Autodesk Fusion 360 part; units mm, degrees
(part 2 of 2)
sketch "SDVX Layout" plane through (0, 77, 0) normal (0, 1, 0) x (-1, 0, 0)
  circle A0 centre (-230, 0) radius 2.5
  circle A1 centre (230, 110) radius 2.5
  circle A2 centre (-230, -110) radius 2.5
  circle A3 centre (-230, 110) radius 2.5
  circle A4 centre (0, 110) radius 2.5
  circle A5 centre (230, -110) radius 2.5
  circle A6 centre (0, -110) radius 2.5
  circle A7 centre (230, 0) radius 2.5
  line L0 (-248, 128) -> (-248, -128)
  line L1 (-248, -128) -> (248, -128)
  line L2 (248, -128) -> (248, 128)
  line L3 (248, 128) -> (-248, 128)
  line L4 (248, 0) -> (-248, 0) construction
  line L5 (-151.5, -36) -> (151.5, -36)
  line L6 (67, 28.5) -> (67, -28.5)
  line L7 (-54.5, 62.5) -> (-100.5, 62.5)
  line L8 (-84.5, 31) -> (-146.5, 31) construction
  circle A8 centre (192.49, -61.5) radius 1.75
  circle A9 centre (-179.5, -39) radius 1.75
  line L9 (-47.5, 55.5) -> (-107.5, 98.5) construction
  circle A10 centre (179.5, -54) radius 15 construction
  circle A11 centre (179.5, -54) radius 10
  circle A12 centre (179.5, -54) radius 20
  line L10 (144, -28.5) -> (87, -28.5)
  line L11 (107.5, 55.5) -> (107.5, 98.5)
  line L12 (144, 28.5) -> (144, -28.5)
  line L13 (69.5, -31) -> (69.5, 31) construction
  line L14 (-87, 0) -> (-144, 0) construction
  line L15 (84.5, -31) -> (146.5, 31) construction
  line L16 (-107.5, 55.5) -> (-47.5, 55.5)
  line L17 (146.5, -31) -> (84.5, 31) construction
  line L18 (-54.5, 77) -> (-100.5, 77) construction
  line L19 (67, 0) -> (87, 0) construction
  line L20 (87, 28.5) -> (144, 28.5)
  line L21 (-52.5, 60.5) -> (-102.5, 93.5) construction
  circle A13 centre (179.5, -39) radius 1.75
  line L22 (47.5, 55.5) -> (107.5, 55.5)
  line L23 (144, 0) -> (87, 0) construction
  line L24 (151.5, -36) -> (151.5, 36)
  line L25 (-87, -28.5) -> (-144, -28.5)
  circle A14 centre (-192.49, -61.5) radius 1.75
  circle A15 centre (166.51, -61.5) radius 1.75
  line L26 (84.5, -31) -> (146.5, -31) construction
  line L27 (-84.5, -31) -> (-84.5, 31) construction
  line L28 (52.5, 93.5) -> (52.5, 60.5) construction
  circle A16 centre (-179.5, -54) radius 15 construction
  line L29 (107.5, 98.5) -> (47.5, 98.5)
  line L30 (-47.5, 98.5) -> (-107.5, 98.5)
  line L31 (-102.5, 60.5) -> (-52.5, 60.5) construction
  line L32 (-102.5, 60.5) -> (-52.5, 93.5) construction
  line L33 (-100.5, 62.5) -> (-100.5, 91.5)
  line L34 (100.5, 91.5) -> (100.5, 62.5)
  line L35 (-146.5, 31) -> (-146.5, -31) construction
  line L36 (54.5, 62.5) -> (54.5, 91.5)
  line L37 (52.5, 60.5) -> (102.5, 93.5) construction
  line L38 (-146.5, -31) -> (-84.5, 31) construction
  circle A17 centre (-179.5, -54) radius 10
  line L39 (-146.5, -31) -> (-84.5, -31) construction
  line L40 (47.5, 55.5) -> (107.5, 98.5) construction
  line L41 (107.5, 55.5) -> (47.5, 98.5) construction
  line L42 (-115.5, -28.5) -> (-115.5, 28.5) construction
  line L43 (-84.5, -31) -> (-146.5, 31) construction
  circle A18 centre (-179.5, -54) radius 20
  line L44 (-144, 28.5) -> (-87, 28.5)
  line L45 (54.5, 91.5) -> (100.5, 91.5)
  line L46 (100.5, 62.5) -> (54.5, 62.5)
  line L47 (102.5, 93.5) -> (52.5, 93.5) construction
  line L48 (77.5, 62.5) -> (77.5, 91.5) construction
  line L49 (100.5, 77) -> (54.5, 77) construction
  line L50 (146.5, 31) -> (84.5, 31) construction
  line L51 (-151.5, 36) -> (-151.5, -36)
  line L52 (-107.5, 98.5) -> (-107.5, 55.5)
  line L53 (102.5, 60.5) -> (102.5, 93.5) construction
  circle A19 centre (-166.51, -61.5) radius 1.75
  line L54 (-144, -28.5) -> (-144, 28.5)
  line L55 (-102.5, 93.5) -> (-102.5, 60.5) construction
  line L56 (-87, 28.5) -> (-87, -28.5)
  line L57 (102.5, 60.5) -> (52.5, 93.5) construction
  line L58 (47.5, 98.5) -> (47.5, 55.5)
  line L59 (52.5, 60.5) -> (102.5, 60.5) construction
  line L60 (-10, 0) -> (-67, 0) construction
  line L61 (-7.5, -31) -> (-7.5, 31) construction
  line L62 (7.5, -31) -> (69.5, -31) construction
  line L63 (115.5, -28.5) -> (115.5, 28.5) construction
  line L64 (-100.5, 91.5) -> (-54.5, 91.5)
  line L65 (84.5, 31) -> (84.5, -31) construction
  line L66 (87, -28.5) -> (87, 28.5)
  line L67 (-107.5, 55.5) -> (-47.5, 98.5) construction
  line L68 (38.5, -28.5) -> (38.5, 28.5) construction
  line L69 (146.5, -31) -> (146.5, 31) construction
  line L70 (-87, 0) -> (-67, 0) construction
  line L71 (67, 0) -> (10, 0) construction
  line L72 (151.5, 36) -> (-151.5, 36)
  line L73 (67, -28.5) -> (10, -28.5)
  line L74 (151.5, -36) -> (-151.5, 36) construction
  line L75 (-151.5, -36) -> (151.5, 36) construction
  line L76 (-52.5, 93.5) -> (-102.5, 93.5) construction
  line L77 (52.5, 77) -> (-52.5, 77) construction
  line L78 (10, 28.5) -> (67, 28.5)
  line L79 (-7.5, -31) -> (-69.5, 31) construction
  line L80 (-67, 28.5) -> (-10, 28.5)
  line L81 (7.5, -31) -> (69.5, 31) construction
  line L82 (-47.5, 55.5) -> (-47.5, 98.5)
  line L83 (10, -28.5) -> (10, 28.5)
  line L84 (-7.5, 31) -> (-69.5, 31) construction
  line L85 (-69.5, -31) -> (-7.5, -31) construction
  line L86 (-67, -28.5) -> (-67, 28.5)
  line L87 (-69.5, 31) -> (-69.5, -31) construction
  line L88 (-69.5, -31) -> (-7.5, 31) construction
  line L89 (-10, 28.5) -> (-10, -28.5)
  line L90 (10, 0) -> (-10, 0) construction
  line L91 (-77.5, 62.5) -> (-77.5, 91.5) construction
  line L92 (-52.5, 60.5) -> (-52.5, 93.5) construction
  line L93 (7.5, 31) -> (7.5, -31) construction
  line L94 (-38.5, -28.5) -> (-38.5, 28.5) construction
  circle A20 centre (208, -108) radius 2.5
  line L95 (-10, -28.5) -> (-67, -28.5)
  line L96 (-54.5, 91.5) -> (-54.5, 62.5)
  line L97 (69.5, 31) -> (7.5, 31) construction
  line L98 (69.5, -31) -> (7.5, 31) construction
  line L99 (0, -96.3345) -> (23.3345, -73)
  line L100 (23.3345, -73) -> (0, -49.6655)
  line L101 (0, -49.6655) -> (-23.3345, -73)
  line L102 (-23.3345, -73) -> (0, -96.3345)
  line L103 (0, -96.3345) -> (0, -49.6655) construction
  line L104 (23.3345, -73) -> (-23.3345, -73) construction
  line L105 (0, -128) -> (0, 128) construction
  line L106 (0, -93.2233) -> (20.2233, -73)
  line L107 (20.2233, -73) -> (0, -52.7767)
  line L108 (0, -52.7767) -> (-20.2233, -73)
  line L109 (-20.2233, -73) -> (0, -93.2233)
  line L110 (0, -93.2233) -> (0, -52.7767) construction
  line L111 (20.2233, -73) -> (-20.2233, -73) construction
  point P0 (-10, 0)
  point P1 (10, 0)
  point P2 (87, 0)
  point P3 (-87, 0)
  point P4 (77.5, 62.5)
  point P5 (-77.5, 62.5)
  point P6 (115.5, 0)
  point P7 (-115.5, 0)
  point P8 (38.5, 0)
  point P9 (-38.5, 0)
  point P10 (77.5, 77)
  point P11 (-77.5, 77)
  point P12 (0, 77)
  point P13 (0, -92)
  point P14 (0, -92)
  point P15 (-77.5, 77)
  point P16 (77.5, 77)
  point P17 (0, -96.3345)
  point P18 (0, -73)
  point P19 (0, -73)
  dimension "d218" = 57
  dimension "d219" = 57
  dimension "d220" = 57
  dimension "d221" = 57
  dimension "d222" = 57
  dimension "d223" = 57
  dimension "d224" = 57
  dimension "d225" = 57
  dimension "d227" = 46
  dimension "d228" = 29
  dimension "d229" = 46
  dimension "d230" = 29
  dimension "d231" = 34
  dimension "d238" = 62
  dimension "d239" = 62
  dimension "d240" = 62
  dimension "d241" = 62
  dimension "d242" = 62
  dimension "d243" = 62
  dimension "d244" = 62
  dimension "d245" = 62
  dimension "d246" = 15
  dimension "d247" = 293
  dimension "d248" = 30
  dimension "d249" = 33
  dimension "d250" = 23
  dimension "d251" = 30
  dimension "d252" = 33
  dimension "d253" = 50
  dimension "d254" = 33
  dimension "d255" = 50
  dimension "d256" = 33
  dimension "d258" = 105
  dimension "d259" = 20
  dimension "d260" = 20
  dimension "d267" = 61
  dimension "d268" = 5
  dimension "d269" = 5
  dimension "d270" = 5
  dimension "d271" = 5
  dimension "d272" = 5
  dimension "d273" = 5
  dimension "d274" = 3.5
  dimension "d275" = 3.5
  dimension "d276" = 3.5
  dimension "d277" = 12.99
  dimension "d278" = 12.99
  dimension "d279" = 7.5
  dimension "d280" = 7.5
  dimension "d281" = 15
  dimension "d282" = 3.5
  dimension "d283" = 3.5
  dimension "d284" = 3.5
  dimension "d285" = 7.5
  dimension "d286" = 7.5
  dimension "d287" = 12.99
  dimension "d288" = 12.99
  dimension "d289" = 15
  dimension "d290" = 40
  dimension "d291" = 40
  dimension "d294" = 33
  dimension "d295" = 33
  dimension "d296" = 55
  dimension "d299" = 28.6
  dimension "d300" = 28.6
  constraint midpoint L2 L4.start
  constraint midpoint L0 L4.end
  constraint horizontal L10
  constraint vertical L66
  constraint horizontal L20
  constraint vertical L12
  constraint horizontal L73
  constraint vertical L83
  constraint horizontal L78
  constraint vertical L6
  constraint horizontal L95
  constraint vertical L86
  constraint horizontal L80
  constraint vertical L89
  constraint horizontal L25
  constraint vertical L54
  constraint horizontal L44
  constraint vertical L56
  constraint midpoint P1 L83
  constraint horizontal origin P1
  constraint midpoint P0 L89
  constraint horizontal P0 origin
  constraint midpoint P3 L56
  constraint horizontal origin P3
  constraint midpoint P2 L66
  constraint horizontal origin P2
  constraint midpoint L23.start L12
  constraint midpoint L14.end L54
  constraint coincident P3 L14.start
  constraint midpoint L60.end L86
  constraint coincident P1 L71.end
  constraint coincident P0 L60.start
  constraint midpoint L19.start L6
  constraint coincident P2 L19.end
  constraint equal L19 L70
  constraint equal L70 L90
  constraint horizontal L46
  constraint vertical L36
  constraint horizontal L45
  constraint vertical L34
  constraint horizontal L7
  constraint vertical L33
  constraint horizontal L64
  constraint vertical L96
  constraint midpoint P4 L46
  constraint midpoint P5 L7
  constraint horizontal P4 P5
  constraint midpoint L49.end L36
  constraint midpoint L18.start L96
  constraint midpoint L63.start L10
  constraint midpoint L63.end L20
  constraint midpoint L68.start L73
  constraint midpoint L68.end L78
  constraint midpoint L94.start L95
  constraint midpoint L94.end L80
  constraint midpoint L42.start L25
  constraint midpoint L42.end L44
  constraint horizontal L26
  constraint perpendicular L26 L69
  constraint parallel L26 L50
  constraint parallel L65 L69
  constraint coincident P6 L15
  constraint coincident P6 L17
  constraint midpoint P6 L23
  constraint horizontal L62
  constraint perpendicular L13 L62
  constraint parallel L62 L97
  constraint parallel L13 L93
  constraint coincident P8 L81
  constraint coincident P8 L98
  constraint midpoint P8 L71
  constraint horizontal L85
  constraint perpendicular L61 L85
  constraint parallel L84 L85
  constraint parallel L61 L87
  constraint coincident P9 L88
  constraint coincident P9 L79
  constraint midpoint P9 L60
  constraint horizontal L39
  constraint perpendicular L27 L39
  constraint parallel L8 L39
  constraint parallel L27 L35
  constraint coincident P7 L38
  constraint coincident P7 L43
  constraint midpoint P7 L42
  constraint horizontal A16.centre A10.centre
  constraint midpoint L49.start L34
  constraint midpoint L18.end L33
  constraint coincident P4 L48.start
  constraint midpoint L48.end L45
  constraint coincident P5 L91.start
  constraint midpoint L91.end L64
  constraint horizontal L59
  constraint perpendicular L53 L59
  constraint parallel L47 L59
  constraint parallel L28 L53
  constraint coincident P16 L37
  constraint coincident P16 L57
  constraint midpoint P16 L49
  constraint horizontal L31
  constraint perpendicular L31 L92
  constraint parallel L31 L76
  constraint parallel L55 L92
  constraint coincident P15 L32
  constraint coincident P15 L21
  constraint midpoint P15 L91
  constraint midpoint L77.start L28
  constraint midpoint L77.end L92
  constraint midpoint P12 L77
  constraint vertical origin P12
  constraint concentric A10 A11
  constraint concentric A16 A17
  constraint coincident P14 P13
  constraint vertical origin P14
  constraint horizontal L5
  constraint perpendicular L5 L24
  constraint parallel L5 L72
  constraint parallel L24 L51
  constraint coincident origin L75
  constraint coincident origin L74
  constraint horizontal L22
  constraint perpendicular L11 L22
  constraint parallel L22 L29
  constraint parallel L11 L58
  constraint coincident P16 L40
  constraint coincident P16 L41
  constraint coincident P16 P10
  constraint horizontal L16
  constraint perpendicular L16 L82
  constraint parallel L16 L30
  constraint parallel L52 L82
  constraint coincident P15 L67
  constraint coincident P15 L9
  constraint coincident P15 P11
  constraint vertical A10.centre A13.centre
  constraint vertical A16.centre A9.centre
  constraint concentric A10 A12
  constraint concentric A17 A18
  constraint perpendicular L99 L100
  constraint parallel L99 L101
  constraint parallel L100 L102
  constraint coincident L103 P19
  constraint coincident L104 P19
  constraint coincident P17 L99.start
  constraint midpoint L1 L105.start
  constraint midpoint L3 L105.end
  constraint coincident P19 L105
  constraint perpendicular L106 L107
  constraint parallel L106 L108
  constraint parallel L107 L109
  constraint coincident L110 P19
  constraint coincident L111 P19
  constraint coincident P19 P18
  measures "d218" distance of L10.start L10.end
  measures "d219" distance of L10.start L12.start
  measures "d220" distance of L73.end L6.end
  measures "d221" distance of L6.start L6.end
  measures "d222" distance of L89.end L86.start
  measures "d223" distance of L80.end L89.end
  measures "d224" distance of L25.start L44.end
  measures "d225" distance of L25.start L25.end
  measures "d227" distance of L34.end L36.start
  measures "d228" distance of L34.end L34.start
  measures "d229" distance of L7.start L7.end
  measures "d230" distance of L7.start L64.end
  measures "d231" distance of L46 L78
  measures "d238" distance of L15.end L17.end
  measures "d239" distance of L17.start L15.end
  measures "d240" distance of L93.start L13.end
  measures "d241" distance of L13.end L13.start
  measures "d242" distance of L61.end L79.end
  measures "d243" distance of L61.start L61.end
  measures "d244" distance of L8.start L8.end
  measures "d245" distance of L8.start L27.start
  measures "d246" distance of L13 L65
  measures "d247" distance of L35 L69
  measures "d248" diameter of A10
  measures "d249" distance of A10.centre L69
  measures "d250" distance of A10.centre L26
  measures "d251" diameter of A16
  measures "d252" distance of A16.centre L35
  measures "d253" distance of L28.start L37.end
  measures "d254" distance of L37.end L53.start
  measures "d255" distance of L32.end L21.end
  measures "d256" distance of L32.end L21.start
  measures "d258" distance of L77.start L77.end
  measures "d259" diameter of A11
  measures "d260" diameter of A17
  measures "d267" distance of P14 L85
  measures "d268" distance of L24 L69
  measures "d269" distance of L5 L26
  measures "d270" distance of L22 L59
  measures "d271" distance of L11 L53
  measures "d272" distance of L16 L31
  measures "d273" distance of L52 L55
  measures "d274" diameter of A8
  measures "d275" diameter of A15
  measures "d276" diameter of A13
  measures "d277" horizontal distance of A10.centre A8.centre
  measures "d278" horizontal distance of A10.centre A15.centre
  measures "d279" vertical distance of A10.centre A8.centre
  measures "d280" vertical distance of A10.centre A15.centre
  measures "d281" vertical distance of A10.centre A13.centre
  measures "d282" diameter of A19
  measures "d283" diameter of A14
  measures "d284" diameter of A9
  measures "d285" vertical distance of A16.centre A19.centre
  measures "d286" vertical distance of A16.centre A14.centre
  measures "d287" horizontal distance of A16.centre A19.centre
  measures "d288" horizontal distance of A16.centre A14.centre
  measures "d289" vertical distance of A16.centre A9.centre
  measures "d290" diameter of A12
  measures "d291" diameter of A18
  measures "d294" distance of L100.end L101.end
  measures "d295" distance of L99.end L100.end
  measures "d296" distance of L1 P19
  measures "d299" distance of L107.end L108.end
  measures "d300" distance of L106.end L107.end
extrude "Extrude24" cut sketch "SDVX Layout" against normal up to surface (9 mm away) contours L6 L73 L78 L83 | L7 L33 L64 L96 | A8 | A9 | A11 | L10 L12 L20 L66 | A13 | L25 L44 L54 L56 | A14 | A15 | L34 L36 L45 L46 | A17 | A19 | L80 L86 L89 L95 | L106 L107 L108 L109 bodies 3 8 in component "Box"
extrude "Extrude25" cut sketch "SDVX Layout" against normal up to surface (9 mm away) contours L5 L24 L51 L72 | A12 | L11 L22 L29 L58 | L16 L30 L52 L82 | A18 | L99 L100 L101 L102 bodies 3 in component "Box"
sketch "USB panel" plane through (0, 0, -128) normal (0, 0, -1) x (-1, 0, 0)
  circle A0 centre (0, 60) radius 2.5
  circle A1 centre (231, 60) radius 2.5
  circle A2 centre (-231, 60) radius 2.5
  circle A3 centre (0, 14) radius 2.5
  circle A4 centre (231, 14) radius 2.5
  circle A5 centre (-231, 14) radius 2.5
  line L0 (-245, 74) -> (-245, 0)
  line L1 (-245, 0) -> (245, 0)
  line L2 (245, 0) -> (245, 74)
  line L3 (245, 74) -> (-245, 74)
  line L4 (6.5, 35.5) -> (-6.5, 35.5)
  line L5 (-6.5, 35.5) -> (-6.5, 22.5)
  line L6 (-6.5, 22.5) -> (6.5, 22.5)
  line L7 (6.5, 22.5) -> (6.5, 35.5)
  line L8 (6.5, 35.5) -> (-6.5, 22.5) construction
  line L9 (-6.5, 35.5) -> (6.5, 22.5) construction
  circle A6 centre (-13, 29) radius 1.6
  circle A7 centre (13, 29) radius 1.6
  line L10 (-13, 29) -> (13, 29) construction
  line L11 (0, 74) -> (0, 0) construction
  line L12 (20, 38.5) -> (-20, 38.5)
  line L13 (-20, 38.5) -> (-20, 19.5)
  line L14 (-20, 19.5) -> (20, 19.5)
  line L15 (20, 19.5) -> (20, 38.5)
  line L16 (20, 38.5) -> (-20, 19.5) construction
  line L17 (-20, 38.5) -> (20, 19.5) construction
  point P0 (0, 29)
  point P1 (0, 29)
  dimension "d305" = 13
  dimension "d306" = 13
  dimension "d307" = 3.2
  dimension "d308" = 3.2
  dimension "d309" = 6.5
  dimension "d310" = 6.5
  dimension "d311" = 6.5
  dimension "d312" = 6.5
  dimension "d313" = 29
  dimension "d314" = 40
  dimension "d315" = 19
  constraint horizontal L4
  constraint perpendicular L4 L5
  constraint parallel L4 L6
  constraint parallel L5 L7
  constraint coincident L8 P1
  constraint coincident L9 P1
  constraint coincident A6.centre L10.start
  constraint coincident A7.centre L10.end
  constraint midpoint L3 L11.start
  constraint coincident L11.end origin
  constraint vertical P1 L11.start
  constraint horizontal L12
  constraint perpendicular L12 L13
  constraint parallel L12 L14
  constraint parallel L13 L15
  constraint coincident L16 P1
  constraint coincident L17 P1
  constraint coincident P1 P0
  measures "d305" distance of L5.end L6.end
  measures "d306" distance of L4.end L5.end
  measures "d307" diameter of A6
  measures "d308" diameter of A7
  measures "d309" distance of L5 A6.centre
  measures "d310" distance of L7 A7.centre
  measures "d311" distance of L4 A6.centre
  measures "d312" distance of L4 A7.centre
  measures "d313" distance of L1 P1
  measures "d314" distance of L13.end L14.end
  measures "d315" distance of L12.end L13.end
extrude "Extrude26" cut sketch "USB panel" against normal up to surface (9 mm away) contours L4 L5 L6 L7 | A6 | A7 bodies 4 12 in component "Box"
extrude "Extrude27" cut sketch "USB panel" against normal up to surface (9 mm away) contours L12 L13 L14 L15 bodies 4 in component "Box"
extrude "Extrude6" [suppressed] in component "Box"
pattern_linear "R-Pattern4" [suppressed] in component "Box"
pattern_linear "R-Pattern5" [suppressed] in component "Box"
component "Box" placed x (1, 0, 0) y (0, 1, 0) z (0, 0, 1) at (0, 0, 0)
equation "length = 490 mm" comment "X axis"
equation "width = 250 mm" comment "Y axis"
equation "height = 74 mm" comment "Z axis"
equation "thickness = 6 mm"
equation "ciLength = length - thickness * 2" comment "Calculated Inner Length"
equation "ciWidth = width - thickness * 2" comment "Calculated Inner Width"
equation "ciHeight = height - thickness" comment "Calculated Inner Height"
equation "fingerw = thickness * 2" comment "Optimal finger Width"
equation "lfingers = max(3; ( floor(ceil(length / fingerw) / 2) * 2 ) - 1)" comment "Length axis: Number of fingers"
equation "lfingerw = length / lfingers" comment "Length axis: Actual finger width"
equation "lnotches = floor(lfingers / 2)" comment "Length axis: Number of notches along the edge"
equation "lnotchl = ( lfingers - 2 ) * lfingerw" comment "Length axis: Length of the notch reference line"
equation "hfingers = max(3; ( floor(ceil(ciHeight / fingerw) / 2) * 2 ) - 1)" comment "Height axis: Number of fingers"
equation "hfingerw = height / hfingers" comment "Height axis: Actual finger width"
equation "hnotches = floor(hfingers / 2)" comment "Height axis: Number of notches along the edge"
equation "hnotchl = ( hfingers - 2 ) * hfingerw" comment "Height axis: Length of the notch reference line"
equation "wfingers = max(3; ( floor(ceil(width / fingerw) / 2) * 2 ) - 1)" comment "Width axis: Number of fingers"
equation "wfingerw = width / wfingers" comment "Width axis: Actual finger width"
equation "wnotches = floor(wfingers / 2)" comment "Width axis: Number of notches along the edge"
equation "wnotchl = ( wfingers - 2 ) * wfingerw" comment "Width axis: Length of the notch reference line"
equation "d31 = length"
equation "d32 = width"
equation "d33 = thickness"
equation "d35 = lfingerw"
equation "d36 = lnotchl"
equation "d37 = -thickness"
equation "d39 = lnotches"
equation "d41 = ( lnotchl - lfingerw ) * -1"
equation "d42 = width - thickness"
equation "d43 = wfingerw"
equation "d44 = wnotchl"
equation "d45 = -thickness"
equation "d47 = wnotches"
equation "d49 = ( wnotchl - wfingerw ) * -1"
equation "d50 = length - thickness"
equation "d51 = length"
equation "d52 = height"
equation "d53 = -thickness"
equation "d55 = thickness"
equation "d56 = hfingerw"
equation "d57 = hnotchl"
equation "d58 = -thickness"
equation "d60 = hnotches"
equation "d62 = ( hnotchl - hfingerw ) * -1"
equation "d63 = ( length - thickness ) * -1"
equation "d66 = -thickness"
equation "d68 = lnotches"
equation "d70 = lnotchl - lfingerw"
equation "d74 = ( width - thickness ) * -1"
equation "d82 = height - thickness"
equation "d86 = ( width - thickness ) * -1"
equation "d88 = width"
equation "d89 = height"
equation "d90 = -thickness"
equation "d94 = length - thickness"
equation "aThickness = 3 mm" comment "Outer Acrylic Plates Thickness"
equation "aScrew = 5 mm" comment "Outer Acrylic screws hole diameter"
equation "d100 = length + aThickness * 2"
equation "d101 = width + aThickness * 2"
equation "d102 = -aThickness"
equation "d106 = height + aThickness"
equation "d115 = height"
equation "d116 = width"
equation "d117 = height"
equation "d118 = width + aThickness * 2"
equation "d119 = aThickness"
equation "d123 = length + aThickness"
equation "d125 = height"
equation "d126 = length"
equation "d127 = length"
equation "d128 = height"
equation "d129 = width / 2"
equation "d130 = aThickness"
equation "d134 = ( width + aThickness ) * -1"
equation "d136 = aScrew"
equation "d137 = aThickness + thickness + aScrew + 4 mm"
equation "d138 = aThickness + thickness + aScrew + 4 mm"
equation "d141 = -length + ( aThickness + thickness + aScrew ) * 2 - thickness + 8 mm"
equation "d142 = width - ( aThickness + thickness + aScrew ) * 2 + thickness - 8 mm"
equation "d143 = -aThickness - thickness"
equation "d145 = -height - thickness"
equation "d146 = thickness + aThickness"
equation "d148 = aScrew"
equation "d149 = aScrew + aThickness + thickness"
equation "d150 = aScrew + aThickness + thickness + 4 mm"
equation "d151 = height"
equation "d152 = width + aThickness * 2"
equation "d155 = width - ( aScrew + aThickness + thickness ) * 2 + thickness - 8 mm"
equation "d156 = ( height - ( aScrew + aThickness + thickness ) * 2 ) * -1"
equation "d159 = aScrew"
equation "d160 = aScrew + aThickness + thickness"
equation "d161 = aScrew + aThickness + thickness"
equation "d164 = length - ( aScrew + aThickness + thickness ) * 2"
equation "d165 = ( height - ( aScrew + aThickness + thickness ) * 2 ) * -1"
equation "d168 = length - ( thickness + aThickness + aScrew ) * 2 - thickness - 15 mm"
equation "d169 = width - ( thickness + aThickness + aScrew ) * 2 - thickness - 15 mm"
equation "d170 = -thickness"
equation "d192 = -aThickness"
equation "d199 = width - ( aScrew + aThickness + thickness ) * 2 + thickness - 8 mm"
equation "d200 = ( height - ( aScrew + aThickness + thickness ) * 2 ) * -1"
equation "d205 = -length + ( aThickness + thickness + aScrew ) * 2 - thickness + 8 mm"
equation "d206 = width - ( aThickness + thickness + aScrew ) * 2 + thickness - 8 mm"
equation "d249 = ( 30 / 2 ) * 1 mm + 18 mm"
equation "d252 = ( 30 / 2 ) * 1 mm + 18 mm"
equation "d315 = 13 mm + 6 mm"
named bodies: "Bottom Panel", "Front Panel", "Front Panel (1)", "Top Panel", "Back Panel", "Left Panel", "Right Panel", "Bottom Plate", "Top Plate", "Left Plate", "Right Plate", "Front Plate", "Back Plate"
